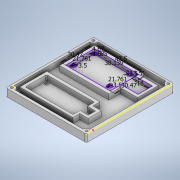
# Autodesk Inventor part: Case 1
Saved by Autodesk Inventor 2020.2 (Build 242310000, 310)
## iProperties
Created: 2019-11-25
Part Number: Case 1
Material: Generic
Document SubType Name: Modeling
Designer: athiy
Density: 1 g/cm^3
Appearance: Default
Author: athiy
Autodesk Inventor part; units mm, degrees
ref_plane "YZ Plane" through (0, 0, 0) normal (1, 0, 0) x (0, 1, 0)
ref_plane "XZ Plane" through (0, 0, 0) normal (0, 1, 0) x (-1, 0, 0)
ref_plane "XY Plane" through (0, 0, 0) normal (0, 0, 1) x (1, 0, 0)
sketch "Sketch1" plane through (0, 0, 0) normal (0, 1, 0) x (-1, 0, 0)
  line L0 (-81.2549, 4.894) -> (-81.2549, -88.547)
  line L1 (4.6415, -88.547) -> (4.6415, 4.894)
  line L2 (4.6415, -88.547) -> (-81.2549, -88.547)
  line L3 (4.6415, 4.894) -> (-81.2549, 4.894)
  point P0 (0, 0)
  constraints: 8 end point, 1 horizontal, 1 perpendicular, 1 vertical
extrude "Extrusion1" add sketch "Sketch1" along normal blind 8
fillet "Fillet1" radius 2 1 edges at (81.2549, 4, -88.547)
sketch "Sketch2" plane through (0, 8, 0) normal (0, 1, 0) x (1, 0, 0)
  line L0 (0, 0) -> (5, 0)
  line L1 (2, 0) -> (76, 0) projected
  line L2 (5, 6) -> (5, 28.88)
  line L3 (5, 28.88) -> (56, 28.88)
  line L4 (56, 28.88) -> (56, 6)
  line L5 (56, 6) -> (5, 6)
  line L6 (0, 83) -> (0, 2) projected
  line L7 (5, 42.5) -> (5, 72.97)
  line L8 (5, 72.97) -> (52.5, 72.97)
  line L9 (52.5, 72.97) -> (52.5, 42.5)
  line L10 (52.5, 42.5) -> (5, 42.5)
  line L11 (5, 6) -> (5, 8.504)
  circle A0 centre (7.54, 8.504) radius 1.27
  line L12 (5, 17.44) -> (56, 17.44)
  line L13 (30.5, 6) -> (30.5, 28.88)
  circle A1 centre (7.54, 26.376) radius 1.27
  circle A2 centre (53.46, 8.504) radius 1.27
  circle A3 centre (53.46, 26.376) radius 1.27
  circle A4 centre (7.54, 8.504) radius 1.7
  circle A5 centre (7.54, 26.376) radius 1.7
  circle A6 centre (53.46, 8.504) radius 1.7
  circle A7 centre (53.46, 26.376) radius 1.7
  circle A8 centre (7.54, 26.376) radius 1.7
  line L14 (56, 17.44) -> (56, 21.34)
  line L15 (56, 17.44) -> (56, 13.54)
  line L16 (56, 13.54) -> (64.7, 13.54)
  line L17 (64.7, 13.54) -> (64.7, 21.34)
  line L18 (64.7, 21.34) -> (56, 21.34)
  dimension "d6" = 6
  dimension "d7" = 22.88
  dimension "d8" = 51
  dimension "d9" = 30.47
  dimension "d10" = 47.5
  dimension "d14" = 2.504
  dimension "d16" = 2.54
  dimension "d17" = 3.4
  dimension "d35" = 8.7
  constraints: 34 end point, 9 centre point, 9 perpendicular, 6 symmetric about line, 4 midpoint, 4 point on line, 2 coincident, 1 concentric, 1 vertical, 6 other
  measures "d6" distance of L0.end L2.start
  measures "d7" distance of L2.start L2.end
  measures "d8" distance of L2.end L3.end
  measures "d9" distance of L7.start L7.end
  measures "d10" distance of L7.end L8.end
  measures "d14" distance of L2.start L11.end
  measures "d16" diameter of A0
  measures "d17" diameter of A4
  measures "d35" distance of L15.end L16.end
extrude "Extrusion2" cut sketch "Sketch2" against normal blind 5.75 contours L2 L12 L13 L5 | L13 L12 L4 L5 | L2 L3 L13 L12 | L13 L3 L4 L12 | L4 L18 L17 L16 | A0 | A1 | A2 | A3 | A4 | A5 | A6 | A7
fillet "Fillet2" radius 1.27 4 edges at (5, 5.125, -28.88) (56, 5.125, -28.88) (5, 5.125, -6) (56, 5.125, -6)
sketch "Sketch3" plane through (0, 2.25, 0) normal (0, 1, 0) x (1, 0, 0)
  point P0 (0, 0)
sketch "Sketch4" plane through (0, 2.25, 0) normal (0, 1, 0) x (1, 0, 0)
  arc A0 (6.27, 28.88) -> (5, 27.61) centre (6.27, 27.61) ccw projected
  line L0 (6.27, 27.61) -> (8.041, 27.61) construction
  circle A1 centre (7.5401, 26.3758) radius 1.27
  line L1 (5, 7.27) -> (5, 27.61) projected
  line L2 (5, 17.44) -> (56, 17.44)
  line L3 (56, 27.61) -> (56, 7.27) projected
  line L4 (6.27, 28.88) -> (54.73, 28.88) projected
  line L5 (6.27, 28.88) -> (30.5, 28.88)
  line L6 (6.27, 28.88) -> (30.5, 28.88) construction
  line L7 (30.5, 28.88) -> (30.5, 0)
  circle A2 centre (7.5401, 8.5042) radius 1.27
  circle A3 centre (53.4599, 26.3758) radius 1.27
  circle A4 centre (53.4599, 8.5042) radius 1.27
  circle A5 centre (7.5401, 26.3758) radius 1.9
  circle A6 centre (53.4599, 26.3758) radius 1.9
  circle A7 centre (7.5401, 8.5042) radius 1.9
  circle A8 centre (53.4599, 8.5042) radius 1.9
  point P0 (0, 0)
  dimension "d21" = 24.23
  dimension "d22" = 0
  dimension "d23" = 90
  dimension "d24" = 3.8
  constraints: 10 end point, 8 centre point, 6 symmetric about line, 2 collinear, 2 horizontal, 2 midpoint, 1 coincident, 6 other
  measures "d21" distance of L4.start L5.end
  measures "d22" distance between parallel lines of L5 L6
  measures "d23" angle of L5 L7
  measures "d24" diameter of A5
extrude "Extrusion3" add sketch "Sketch4" along normal blind 1.4 contours A5 | A6 | A7 | A8
sketch "Sketch5" plane through (7.5401, 2.25, -26.3758) normal (0, 1, 0) x (1, 0, 0)
  circle A0 centre (0, 0) radius 1.27
  point P0 (-7.5401, -26.3758)
  constraints: 1 centre point
extrude "Extrusion4" cut sketch "Sketch5" against normal blind 3
sketch "Sketch6" plane through (7.5401, 2.25, -8.5042) normal (0, 1, 0) x (1, 0, 0)
  circle A0 centre (0, 0) radius 1.9 projected
  circle A1 centre (0, 0) radius 1.27
  point P0 (-7.5401, -8.5042)
  constraints: 1 centre point, 1 coincident
extrude "Extrusion5" cut sketch "Sketch6" against normal blind 3 contours A1
sketch "Sketch7" plane through (53.4599, 2.25, -26.3758) normal (0, 1, 0) x (1, 0, 0)
  circle A0 centre (0, 0) radius 1.27 projected
  circle A1 centre (0, 0) radius 1.27
  point P0 (-53.4599, -26.3758)
  constraints: 1 centre point, 1 coincident
extrude "Extrusion6" cut sketch "Sketch7" against normal blind 3
sketch "Sketch8" plane through (53.4599, 2.25, -8.5042) normal (0, 1, 0) x (1, 0, 0)
  circle A0 centre (0, 0) radius 1.27 projected
  circle A1 centre (0, 0) radius 1.27
  point P0 (-53.4599, -8.5042)
  constraints: 1 centre point, 1 coincident
sketch "Sketch9" plane through (0, 8, 0) normal (0, 1, 0) x (1, 0, 0)
  line L0 (6.27, 47.7819) -> (6.27, 78.2519)
  line L1 (6.27, 78.2519) -> (53.77, 78.2519)
  line L2 (53.77, 78.2519) -> (53.77, 47.7819)
  line L3 (53.77, 47.7819) -> (6.27, 47.7819)
  line L4 (81.2549, -4.894) -> (81.2549, 86.547) projected
  line L5 (53.77, 78.2519) -> (53.77, 74.7519)
  line L6 (53.77, 74.7519) -> (71.77, 74.7519)
  line L7 (71.77, 74.7519) -> (71.77, 59.4972)
  line L8 (71.77, 59.4972) -> (53.77, 59.4972)
  line L9 (6.27, 78.2519) -> (10.94, 78.2519)
  line L10 (10.94, 78.2519) -> (10.94, 73.5819)
  circle A0 centre (10.94, 73.5819) radius 1.75
  line L11 (10.94, 73.5819) -> (10.94, 51.8209)
  circle A1 centre (10.94, 51.8209) radius 1.75
  line L12 (10.94, 73.5819) -> (49.079, 73.5819)
  circle A2 centre (49.079, 73.5819) radius 1.75
  line L13 (49.079, 73.5819) -> (49.079, 51.8209)
  circle A3 centre (49.079, 51.8209) radius 1.75
  circle A4 centre (10.94, 73.5819) radius 2.4749
  circle A5 centre (49.079, 73.5819) radius 2.4749
  circle A6 centre (49.079, 51.8209) radius 2.4749
  circle A7 centre (10.94, 51.8209) radius 2.4749
  point P0 (0, 0)
  point P1 (81.2549, 2)
  dimension "d37" = 30.47
  dimension "d38" = 47.5
  dimension "d39" = 30.47
  dimension "d63" = 3.5
  dimension "d64" = 18
  dimension "d94" = 4.67
  dimension "d95" = 4.67
  dimension "d96" = 3.5
  dimension "d97" = 21.761
  dimension "d98" = 3.5
  dimension "d99" = 38.139
  dimension "d100" = 3.5
  dimension "d101" = 21.761
  dimension "d102" = 3.5
  constraints: 26 end point, 8 centre point, 6 perpendicular, 3 coincident, 3 point on line, 3 vertical, 1 horizontal
  measures "d37" distance of L0.start L0.end
  measures "d38" distance of L0.end L1.end
  measures "d39" distance of L1.end L2.end
  measures "d63" distance of L1.end L5.end
  measures "d64" distance of L5.end L6.end
  measures "d94" distance of L0.end L9.end
  measures "d95" distance of L9.end L10.end
  measures "d96" diameter of A0
  measures "d97" distance of L11.start L11.end
  measures "d98" diameter of A1
  measures "d99" distance of L11.start L12.end
  measures "d100" diameter of A2
  measures "d101" distance of L13.start L13.end
  measures "d102" diameter of A3
extrude "Extrusion7" cut sketch "Sketch9" against normal blind 4.95 contours L0 L1 L2 L3 | L2 L6 L7 L8 | A4 L12 A0 L10 | L10 A0 L11 A4 | A0 L12 L10 | L10 L11 A0 | A4 L11 A0 L12 | L12 A0 L11 | A1 | A5 L13 A2 L12 | L12 A2 L13 A5 | A2 L13 L12 | L12 L13 A2 | A3 | A6 | A7
fillet "Fillet3" radius 1.6 4 edges at (6.27, 5.525, -47.7819) (6.27, 5.525, -78.2519) (53.77, 5.525, -78.2519) (53.77, 5.525, -47.7819)
extrude "Extrusion9" cut sketch "Sketch8" against normal blind 3
sketch "Sketch15" plane through (0, 8, 0) normal (0, 1, 0) x (1, 0, 0)
  point P0 (0, 0)
sketch "Sketch16" plane through (0, 8, 0) normal (0, 1, 0) x (1, 0, 0)
  line L0 (53.77, 74.7519) -> (71.77, 74.7519) projected
  line L1 (53.77, 74.7519) -> (71.77, 74.7519)
  line L2 (71.77, 74.7519) -> (71.77, 59.4972) projected
  line L3 (71.77, 74.7519) -> (71.77, 59.4972)
  line L4 (71.77, 59.4972) -> (53.77, 59.4972) projected
  line L5 (71.77, 59.4972) -> (53.77, 59.4972)
  line L6 (7.87, 81.4816) -> (56.0176, 81.4816)
  line L7 (56.0176, 81.4816) -> (56.0176, 78.2519)
  line L8 (56.0176, 78.2519) -> (74.7894, 78.2519)
  line L9 (74.7894, 78.2519) -> (74.7894, 56.2548)
  line L10 (74.7894, 56.2548) -> (56.0176, 56.2548)
  line L11 (56.0176, 56.2548) -> (56.0176, 44.2349)
  line L12 (56.0176, 44.2349) -> (3.4122, 44.2349)
  line L13 (3.4122, 44.2349) -> (3.4122, 81.4816)
  line L14 (3.4122, 81.4816) -> (7.87, 81.4816)
  line L15 (6.27, 32.121) -> (58.6512, 32.121)
  line L16 (58.6512, 32.121) -> (58.6512, 24.5811)
  line L17 (58.6512, 24.5811) -> (67.5733, 24.5811)
  line L18 (67.5733, 24.5811) -> (67.5733, 10.6323)
  line L19 (67.5733, 10.6323) -> (58.6512, 10.6323)
  line L20 (58.6512, 10.6323) -> (58.6512, 3.0924)
  line L21 (58.6512, 3.0924) -> (2.1021, 3.0924)
  line L22 (2.1021, 3.0924) -> (2.1021, 32.121)
  line L23 (2.1021, 32.121) -> (6.27, 32.121)
  circle A0 centre (-0.8495, 85.0914) radius 1.27
  line L24 (-4.6415, 88.547) -> (-4.6415, -4.894) projected
  line L25 (-4.6415, 41.8265) -> (81.2549, 41.8265)
  line L26 (81.2549, -4.894) -> (81.2549, 86.547) projected
  circle A1 centre (-0.8495, -1.4384) radius 1.27
  line L27 (-2.1195, 82.1131) -> (-2.1195, 1.3369)
  line L28 (2.1021, 86.547) -> (74.7894, 86.547)
  arc A2 (-2.1195, 82.1131) -> (2.1021, 86.547) centre (-1.6738, 85.9154) ccw
  line L29 (2.1021, -2.1183) -> (74.7894, -2.1183)
  line L30 (78.4154, 82.1131) -> (78.4154, 1.3369)
  arc A3 (74.7894, 86.547) -> (78.4154, 82.1131) centre (80.0457, 87.1459) ccw
  arc A4 (78.4154, 1.3369) -> (74.7894, -2.1183) centre (78.0984, -1.9607) ccw
  arc A5 (2.1021, -2.1183) -> (-2.1195, 1.3369) centre (-1.3126, -1.9838) ccw
  circle A6 centre (78.0984, -1.9607) radius 1.27
  circle A7 centre (78.0984, 85.6137) radius 1.27
  point P0 (0, 0)
  point P1 (79.2549, 88.547)
  constraints: 52 end point, 14 perpendicular, 8 centre point, 8 point on circle, 7 point on line, 5 horizontal, 3 collinear, 2 symmetric about line, 1 coincident, 1 midpoint, 1 parallel, 1 vertical, 2 other
extrude "Extrusion14" cut sketch "Sketch16" against normal blind 5.75 contours L27 A2 L28 A3 L30 L25 | L25 L30 A4 L29 A5 L27
sketch "Sketch17" plane through (0, 8, 0) normal (0, 1, 0) x (1, 0, 0)
  circle A0 centre (-1.6277, -1.7597) radius 1.27
  line L0 (-4.6415, 88.547) -> (-4.6415, -4.894) projected
  line L1 (-4.6415, 41.8265) -> (80.9593, 41.8265)
  circle A1 centre (-1.6277, 85.4127) radius 1.27
  circle A2 centre (78.2293, -1.7597) radius 1.27
  circle A3 centre (78.2293, 85.4127) radius 1.27
  point P0 (0, 0)
  constraints: 4 centre point, 2 end point, 2 symmetric about line, 1 horizontal, 1 midpoint, 2 other
extrude "Extrusion15" cut sketch "Sketch17" against normal blind 2
fillet "Fillet4" radius 1.6 3 edges at (81.2549, 4, 4.894) (-4.6415, 4, -88.547) (-4.6415, 4, 4.894)
sketch "Sketch19" plane through (0, 3.05, 0) normal (0, 1, 0) x (1, 0, 0)
  point P0 (0, 0)
body "Solid1"
